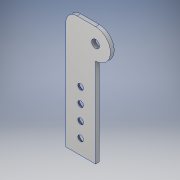
# Autodesk Inventor part: CLB_027_LifterBracketLeft
Saved by Autodesk Inventor 2018.3 (Build 223284000, 284)
## iProperties
Created: 2020-01-12
Part Number: CLB_027_LifterBracketLeft
Material: Aluminum 6061
Document SubType Name: Modeling
Designer: 22perngrac
Density: 2.7 g/cm^3
Appearance: Aluminum - Flat
Author: 22perngrac
Autodesk Inventor part; units mm, degrees
ref_plane "YZ Plane" through (0, 0, 0) normal (1, 0, 0) x (0, 1, 0)
ref_plane "XZ Plane" through (0, 0, 0) normal (0, 1, 0) x (-1, 0, 0)
ref_plane "XY Plane" through (0, 0, 0) normal (0, 0, 1) x (1, 0, 0)
sketch "Sketch1" plane through (0, 0, 0) normal (0, 0, 1) x (1, 0, 0)
  line L0 (0, 0) -> (25.4, 0)
  line L1 (25.4, 0) -> (25.4, 101.6)
  line L2 (25.4, 101.6) -> (0, 101.6)
  line L3 (0, 101.6) -> (0, 0)
  arc A0 (25.4, 76.2) -> (25.4, 101.6) centre (25.4, 88.9) ccw
  dimension "d0" = 101.6
  dimension "d1" = 25.4
  dimension "d2" = 25.4
  constraints: 8 end point, 2 parallel, 2 point on circle, 2 point on line, 1 centre point, 1 horizontal, 1 perpendicular, 1 tangent
  measures "d0" distance of L2.end L0.start
  measures "d1" distance of L0.start L0.end
  measures "d2" diameter of A0
extrude "Extrusion1" add sketch "Sketch1" along normal blind 3.175
sketch "Sketch4" plane through (0, 0, 3.175) normal (0, 0, 1) x (1, 0, 0)
  line L0 (25.4, 0) -> (25.4, 76.2) projected
  arc A0 (25.4, 76.2) -> (25.4, 101.6) centre (25.4, 88.9) ccw projected
  point P0 (0, 0)
  constraints: 1 coincident, 1 point on circle
hole "Hole2" at (25.4, 88.9, 3.175) direction (0, 0, -1) diameter 6.7564 end through all clearance for "Flat Head Machine Screw (82)" size "1/4" standard "Ansi Unified Screw Threads"
fillet "Fillet1" radius 9.525 1 edges at (0, 101.6, 1.5875)
sketch "Sketch6" plane through (0, 0, 0) normal (0, 0, -1) x (-1, 0, 0)
  line L0 (-9.525, 101.6) -> (-25.4, 101.6) projected
  line L1 (0, 92.075) -> (0, 0) projected
  point P0 (-12.7, 50.8)
  dimension "d52" = 50.8
  dimension "d63" = 12.7
  measures "d52" distance from line of L0 point (-12.7, 50.8)
  measures "d63" distance from line of L1 point (-12.7, 50.8)
hole "Hole3" at (12.7, 50.8, 0) direction (0, 0, 1) diameter 4.8514 end through all countersink diameter 9.525 countersink angle 82
pattern_linear "Rectangular Pattern1" count 4 spacing 12.7 along (0, -1, 0) of "Hole3"
equation "\"d2\" = d1"
body "Solid1"
